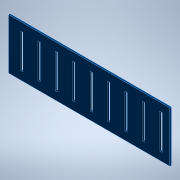
# Autodesk Inventor part: FerriteLayer
Saved by Autodesk Inventor 2021 (Build 250183000, 183)
## iProperties
Created: 2022-02-04
Part Number: FerriteLayer
Material: Generic
Document SubType Name: Modeling
Designer: tlar613
Density: 1 g/cm^3
Appearance: Default
Author: tlar613
Autodesk Inventor part; units mm, degrees
ref_plane "YZ Plane" through (0, 0, 0) normal (1, 0, 0) x (0, 1, 0)
ref_plane "XZ Plane" through (0, 0, 0) normal (0, 1, 0) x (-1, 0, 0)
ref_plane "XY Plane" through (0, 0, 0) normal (0, 0, 1) x (1, 0, 0)
sketch "Sketch1" plane through (0, 0, 0) normal (0, 0, 1) x (1, 0, 0)
  line L0 (-510, 160) -> (510, 160)
  line L1 (510, 160) -> (510, -160)
  line L2 (510, -160) -> (-510, -160)
  line L3 (-510, -160) -> (-510, 160)
  line L4 (0, 224) -> (0, -224) projected
  line L5 (-714, 0) -> (714, 0) projected
  line L6 (5.2, 108.4) -> (20, 108.4)
  line L7 (20, 108.4) -> (20, -108.4)
  line L8 (20, -108.4) -> (5.2, -108.4)
  line L9 (5.2, -108.4) -> (5.2, 108.4)
  line L10 (-104.8, 108.4) -> (-90, 108.4)
  line L11 (-90, 108.4) -> (-90, -108.4)
  line L12 (-90, -108.4) -> (-104.8, -108.4)
  line L13 (-104.8, -108.4) -> (-104.8, 108.4)
  line L14 (-214.8, 108.4) -> (-200, 108.4)
  line L15 (-200, 108.4) -> (-200, -108.4)
  line L16 (-200, -108.4) -> (-214.8, -108.4)
  line L17 (-214.8, -108.4) -> (-214.8, 108.4)
  line L18 (-324.8, 108.4) -> (-310, 108.4)
  line L19 (-310, 108.4) -> (-310, -108.4)
  line L20 (-310, -108.4) -> (-324.8, -108.4)
  line L21 (-324.8, -108.4) -> (-324.8, 108.4)
  line L22 (-434.8, 108.4) -> (-420, 108.4)
  line L23 (-420, 108.4) -> (-420, -108.4)
  line L24 (-420, -108.4) -> (-434.8, -108.4)
  line L25 (-434.8, -108.4) -> (-434.8, 108.4)
  line L26 (115.2, 108.4) -> (130, 108.4)
  line L27 (130, 108.4) -> (130, -108.4)
  line L28 (130, -108.4) -> (115.2, -108.4)
  line L29 (115.2, -108.4) -> (115.2, 108.4)
  line L30 (225.2, 108.4) -> (240, 108.4)
  line L31 (240, 108.4) -> (240, -108.4)
  line L32 (240, -108.4) -> (225.2, -108.4)
  line L33 (225.2, -108.4) -> (225.2, 108.4)
  line L34 (335.2, 108.4) -> (350, 108.4)
  line L35 (350, 108.4) -> (350, -108.4)
  line L36 (350, -108.4) -> (335.2, -108.4)
  line L37 (335.2, -108.4) -> (335.2, 108.4)
  line L38 (460, 108.4) -> (445.2, 108.4)
  line L39 (445.2, 108.4) -> (445.2, -108.4)
  line L40 (445.2, -108.4) -> (460, -108.4)
  line L41 (460, -108.4) -> (460, 108.4)
  point P0 (0, 0)
  dimension "d0" = 1020
  dimension "d1" = 320
  dimension "d2" = 216.8
  dimension "d3" = 14.8
  dimension "d5" = 14.8
  dimension "d8" = 14.8
  dimension "d9" = 14.8
  dimension "d11" = 14.8
  dimension "d14" = 14.8
  dimension "d16" = 14.8
  dimension "d18" = 14.8
  dimension "d20" = 460
  dimension "d21" = 14.8
  dimension "d24" = 110
  dimension "d25" = 110
  dimension "d26" = 110
  dimension "d27" = 110
  dimension "d28" = 110
  dimension "d29" = 110
  dimension "d30" = 110
  dimension "d31" = 110
  constraints: 80 end point, 20 parallel, 15 collinear, 10 horizontal, 10 perpendicular, 4 other
  measures "d0" distance of L0.start L0.end
  measures "d1" distance of L0.end L1.end
  measures "d2" distance of L6.end L7.end
  measures "d3" distance of L6.start L6.end
  measures "d5" distance of L11.end L12.end
  measures "d8" distance of L15.end L16.end
  measures "d9" distance of L19.end L20.end
  measures "d11" distance of L23.end L24.end
  measures "d14" distance of L27.end L28.end
  measures "d16" distance of L31.end L32.end
  measures "d18" distance of L35.end L36.end
  measures "d20" distance between parallel lines of L4 L41
  measures "d21" distance of L39.end L40.end
  measures "d24" distance between parallel lines of L39 L37
  measures "d25" distance between parallel lines of L37 L33
  measures "d26" distance between parallel lines of L33 L29
  measures "d27" distance between parallel lines of L29 L9
  measures "d28" distance between parallel lines of L9 L13
  measures "d29" distance between parallel lines of L13 L17
  measures "d30" distance between parallel lines of L17 L21
  measures "d31" distance between parallel lines of L21 L25
extrude "Extrusion1" add sketch "Sketch1" along normal blind 10 contours L0 L4 L5 L11 L10 L13 L15 L14 L17 L19 L18 L21 L23 L22 L25 L3 | L0 L1 L5 L41 L38 L39 L35 L34 L37 L31 L30 L33 L27 L26 L29 L7 L6 L9 L4 | L5 L25 L24 L23 L21 L20 L19 L17 L16 L15 L13 L12 L11 L4 L2 L3 | L5 L9 L8 L7 L29 L28 L27 L33 L32 L31 L37 L36 L35 L39 L40 L41 L1 L2 L4
body "Solid1"
